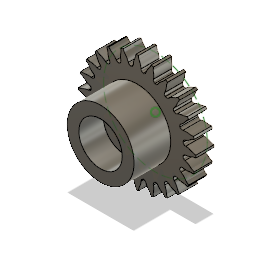
Frame Motor Gear (1) (Autodesk Fusion 360 design; units mm, degrees)
description: Spur Gear; Module: 0.708340; Num Teeth: 24; Pressure Angle: 20.000000; Backlash: 0.00 mm
Autodesk Fusion 360 part; units mm, degrees
(part 1 of 7)
sketch "Sketch1" plane through (0, 0, 0) normal (0, 0, 1) x (1, 0, 0) in component "Spur Gear (24 teeth)"
  circle A0 centre (0, 0) radius 7.5993
  circle A1 centre (0, 0) radius 0.35
extrude "Extrude1" add sketch "Sketch1" along normal blind 3 in component "Spur Gear (24 teeth)"
sketch "Sketch2" plane through (0, 0, 0) normal (0, 0, 1) x (1, 0, 0) in component "Spur Gear (24 teeth)"
  spline S0 degree 5 poles (7.9617, -0.6411) (7.9654, -0.6414) (7.9728, -0.6419) (7.9839, -0.6424) (7.9987, -0.6424) (8.0173, -0.6418) (8.0359, -0.6406) (8.0545, -0.6391) (8.0731, -0.6375) (8.0917, -0.6357) (8.1103, -0.6338) (8.129, -0.6317) (8.1476, -0.6294) (8.1663, -0.6268) (8.185, -0.6239) (8.2036, -0.6208) (8.2223, -0.6175) (8.241, -0.6141) (8.2597, -0.6105) (8.2783, -0.6068) (8.297, -0.6029) (8.3157, -0.5988) (8.3344, -0.5946) (8.3531, -0.5902) (8.3718, -0.5857) (8.3904, -0.581) (8.4091, -0.5761) (8.4278, -0.5711) (8.4465, -0.566) (8.4652, -0.5608) (8.4838, -0.5554) (8.5025, -0.5499) (8.5211, -0.5442) (8.5398, -0.5384) (8.5584, -0.5325) (8.5771, -0.5265) (8.5958, -0.5203) (8.6145, -0.514) (8.6331, -0.5076) (8.6517, -0.5011) (8.6703, -0.4944) (8.6888, -0.4876) (8.7073, -0.4807) (8.7258, -0.4737) (8.7445, -0.4666) (8.7632, -0.4593) (8.782, -0.452) (8.8008, -0.4445) (8.8194, -0.4369) (8.8377, -0.4292) (8.8558, -0.4214) (8.8737, -0.4136) (8.8918, -0.4056) (8.9103, -0.3974) (8.9293, -0.3891) (8.949, -0.3807) (8.9689, -0.3722) (8.9882, -0.3636) (9.0065, -0.3549) (9.0233, -0.3463) (9.0386, -0.3376) (9.0533, -0.3288) (9.0691, -0.3198) (9.0877, -0.3107) (9.1113, -0.3011) (9.1417, -0.291) (9.1804, -0.2805) (9.2285, -0.2692) (9.2868, -0.2574) (9.3557, -0.2448) (9.4356, -0.2316) (9.5085, -0.2204) (9.5681, -0.2117) (9.6101, -0.2058) (9.6316, -0.2028) knots 0 0 0 0 0 0 0.01428571 0.02857143 0.04285714 0.05714286 0.07142857 0.08571429 0.1 0.11428571 0.12857143 0.14285714 0.15714286 0.17142857 0.18571429 0.2 0.21428571 0.22857143 0.24285714 0.25714286 0.27142857 0.28571429 0.3 0.31428571 0.32857143 0.34285714 0.35714286 0.37142857 0.38571429 0.4 0.41428571 0.42857143 0.44285714 0.45714286 0.47142857 0.48571429 0.5 0.51428571 0.52857143 0.54285714 0.55714286 0.57142857 0.58571429 0.6 0.61428571 0.62857143 0.64285714 0.65714286 0.67142857 0.68571429 0.7 0.71428571 0.72857143 0.74285714 0.75714286 0.77142857 0.78571429 0.8 0.81428571 0.82857143 0.84285714 0.85714286 0.87142857 0.88571429 0.9 0.91428571 0.92857143 0.94285714 0.95714286 0.97142857 0.98571429 1 1 1 1 1 1
  spline S1 degree 5 poles (7.9617, 0.6411) (7.9654, 0.6414) (7.9728, 0.6419) (7.9839, 0.6424) (7.9987, 0.6424) (8.0173, 0.6418) (8.0359, 0.6406) (8.0545, 0.6391) (8.0731, 0.6375) (8.0917, 0.6357) (8.1103, 0.6338) (8.129, 0.6317) (8.1476, 0.6294) (8.1663, 0.6268) (8.185, 0.6239) (8.2036, 0.6208) (8.2223, 0.6175) (8.241, 0.6141) (8.2597, 0.6105) (8.2783, 0.6068) (8.297, 0.6029) (8.3157, 0.5988) (8.3344, 0.5946) (8.3531, 0.5902) (8.3718, 0.5857) (8.3904, 0.581) (8.4091, 0.5761) (8.4278, 0.5711) (8.4465, 0.566) (8.4652, 0.5608) (8.4838, 0.5554) (8.5025, 0.5499) (8.5211, 0.5442) (8.5398, 0.5384) (8.5584, 0.5325) (8.5771, 0.5265) (8.5958, 0.5203) (8.6145, 0.514) (8.6331, 0.5076) (8.6517, 0.5011) (8.6703, 0.4944) (8.6888, 0.4876) (8.7073, 0.4807) (8.7258, 0.4737) (8.7445, 0.4666) (8.7632, 0.4593) (8.782, 0.452) (8.8008, 0.4445) (8.8194, 0.4369) (8.8377, 0.4292) (8.8558, 0.4214) (8.8737, 0.4136) (8.8918, 0.4056) (8.9103, 0.3974) (8.9293, 0.3891) (8.949, 0.3807) (8.9689, 0.3722) (8.9882, 0.3636) (9.0065, 0.3549) (9.0233, 0.3463) (9.0386, 0.3376) (9.0533, 0.3288) (9.0691, 0.3198) (9.0877, 0.3107) (9.1113, 0.3011) (9.1417, 0.291) (9.1804, 0.2805) (9.2285, 0.2692) (9.2868, 0.2574) (9.3557, 0.2448) (9.4356, 0.2316) (9.5085, 0.2204) (9.5681, 0.2117) (9.6101, 0.2058) (9.6316, 0.2028) knots 0 0 0 0 0 0 0.01428571 0.02857143 0.04285714 0.05714286 0.07142857 0.08571429 0.1 0.11428571 0.12857143 0.14285714 0.15714286 0.17142857 0.18571429 0.2 0.21428571 0.22857143 0.24285714 0.25714286 0.27142857 0.28571429 0.3 0.31428571 0.32857143 0.34285714 0.35714286 0.37142857 0.38571429 0.4 0.41428571 0.42857143 0.44285714 0.45714286 0.47142857 0.48571429 0.5 0.51428571 0.52857143 0.54285714 0.55714286 0.57142857 0.58571429 0.6 0.61428571 0.62857143 0.64285714 0.65714286 0.67142857 0.68571429 0.7 0.71428571 0.72857143 0.74285714 0.75714286 0.77142857 0.78571429 0.8 0.81428571 0.82857143 0.84285714 0.85714286 0.87142857 0.88571429 0.9 0.91428571 0.92857143 0.94285714 0.95714286 0.97142857 0.98571429 1 1 1 1 1 1
  arc A0 (9.6316, -0.2028) -> (9.6316, 0.2028) centre (0, 0) ccw
  line L0 (7.5648, -0.61) -> (7.9617, -0.6411)
  line L1 (7.5648, 0.61) -> (7.9617, 0.6411)
  line L2 (7.5648, -0.61) -> (7.5648, 0.61)
extrude "Extrude2" add sketch "Sketch2" along normal blind 3 in component "Spur Gear (24 teeth)"
fillet "Fillet1" radius 0.4 2 edges at (7.5747, -0.6108, 1.5) (7.5747, 0.6108, 1.5) in component "Spur Gear (24 teeth)"
pattern_circular "C-Pattern1" count 24 over 360 about axis through (0, 0, 0) along (0, 0, 1) of "Extrude2", "Fillet1" in component "Spur Gear (24 teeth)"
sketch "Sketch3" plane through (0, 0, 0) normal (0, 0, 1) x (1, 0, 0) in component "Spur Gear (24 teeth)"
  circle A0 centre (0, 0) radius 8.5001 construction
sketch "Sketch1 (2)" plane through (0, 0, 3) normal (0, 0, 1) x (1, 0, 0)
  arc A0 (7.5337, -0.9958) -> (7.5348, -0.988) centre (0, 0) ccw
  arc A1 (7.9617, -0.6411) -> (7.5348, -0.988) centre (7.9314, -1.04) ccw
  spline S0 degree 5 poles (7.9617, -0.6411) (7.9654, -0.6414) (7.9728, -0.6419) (7.9839, -0.6424) (7.9987, -0.6424) (8.0173, -0.6418) (8.0359, -0.6406) (8.0545, -0.6391) (8.0731, -0.6375) (8.0917, -0.6357) (8.1103, -0.6338) (8.129, -0.6317) (8.1476, -0.6294) (8.1663, -0.6268) (8.185, -0.6239) (8.2036, -0.6208) (8.2223, -0.6175) (8.241, -0.6141) (8.2597, -0.6105) (8.2783, -0.6068) (8.297, -0.6029) (8.3157, -0.5988) (8.3344, -0.5946) (8.3531, -0.5902) (8.3718, -0.5857) (8.3904, -0.581) (8.4091, -0.5761) (8.4278, -0.5711) (8.4465, -0.566) (8.4652, -0.5608) (8.4838, -0.5554) (8.5025, -0.5499) (8.5211, -0.5442) (8.5398, -0.5384) (8.5584, -0.5325) (8.5771, -0.5265) (8.5958, -0.5203) (8.6145, -0.514) (8.6331, -0.5076) (8.6517, -0.5011) (8.6703, -0.4944) (8.6888, -0.4876) (8.7073, -0.4807) (8.7258, -0.4737) (8.7445, -0.4666) (8.7632, -0.4593) (8.782, -0.452) (8.8008, -0.4445) (8.8194, -0.4369) (8.8377, -0.4292) (8.8558, -0.4214) (8.8737, -0.4136) (8.8918, -0.4056) (8.9103, -0.3974) (8.9293, -0.3891) (8.949, -0.3807) (8.9689, -0.3722) (8.9882, -0.3636) (9.0065, -0.3549) (9.0233, -0.3463) (9.0386, -0.3376) (9.0533, -0.3288) (9.0691, -0.3198) (9.0877, -0.3107) (9.1113, -0.3011) (9.1417, -0.291) (9.1804, -0.2805) (9.2285, -0.2692) (9.2868, -0.2574) (9.3557, -0.2448) (9.4356, -0.2316) (9.5085, -0.2204) (9.5681, -0.2117) (9.6101, -0.2058) (9.6316, -0.2028) knots 0 0 0 0 0 0 0.01428571 0.02857143 0.04285714 0.05714286 0.07142857 0.08571429 0.1 0.11428571 0.12857143 0.14285714 0.15714286 0.17142857 0.18571429 0.2 0.21428571 0.22857143 0.24285714 0.25714286 0.27142857 0.28571429 0.3 0.31428571 0.32857143 0.34285714 0.35714286 0.37142857 0.38571429 0.4 0.41428571 0.42857143 0.44285714 0.45714286 0.47142857 0.48571429 0.5 0.51428571 0.52857143 0.54285714 0.55714286 0.57142857 0.58571429 0.6 0.61428571 0.62857143 0.64285714 0.65714286 0.67142857 0.68571429 0.7 0.71428571 0.72857143 0.74285714 0.75714286 0.77142857 0.78571429 0.8 0.81428571 0.82857143 0.84285714 0.85714286 0.87142857 0.88571429 0.9 0.91428571 0.92857143 0.94285714 0.95714286 0.97142857 0.98571429 1 1 1 1 1 1
  arc A2 (9.6316, -0.2028) -> (9.6316, 0.2028) centre (0, 0) ccw
  spline S1 degree 5 poles (9.6316, 0.2028) (9.6101, 0.2058) (9.5681, 0.2117) (9.5085, 0.2204) (9.4356, 0.2316) (9.3557, 0.2448) (9.2868, 0.2574) (9.2285, 0.2692) (9.1804, 0.2805) (9.1417, 0.291) (9.1113, 0.3011) (9.0877, 0.3107) (9.0691, 0.3198) (9.0533, 0.3288) (9.0386, 0.3376) (9.0233, 0.3463) (9.0065, 0.3549) (8.9882, 0.3636) (8.9689, 0.3722) (8.949, 0.3807) (8.9293, 0.3891) (8.9103, 0.3974) (8.8918, 0.4056) (8.8737, 0.4136) (8.8558, 0.4214) (8.8377, 0.4292) (8.8194, 0.4369) (8.8008, 0.4445) (8.782, 0.452) (8.7632, 0.4593) (8.7445, 0.4666) (8.7258, 0.4737) (8.7073, 0.4807) (8.6888, 0.4876) (8.6703, 0.4944) (8.6517, 0.5011) (8.6331, 0.5076) (8.6145, 0.514) (8.5958, 0.5203) (8.5771, 0.5265) (8.5584, 0.5325) (8.5398, 0.5384) (8.5211, 0.5442) (8.5025, 0.5499) (8.4838, 0.5554) (8.4652, 0.5608) (8.4465, 0.566) (8.4278, 0.5711) (8.4091, 0.5761) (8.3904, 0.581) (8.3718, 0.5857) (8.3531, 0.5902) (8.3344, 0.5946) (8.3157, 0.5988) (8.297, 0.6029) (8.2783, 0.6068) (8.2597, 0.6105) (8.241, 0.6141) (8.2223, 0.6175) (8.2036, 0.6208) (8.185, 0.6239) (8.1663, 0.6268) (8.1476, 0.6294) (8.129, 0.6317) (8.1103, 0.6338) (8.0917, 0.6357) (8.0731, 0.6375) (8.0545, 0.6391) (8.0359, 0.6406) (8.0173, 0.6418) (7.9987, 0.6424) (7.9839, 0.6424) (7.9728, 0.6419) (7.9654, 0.6414) (7.9617, 0.6411) knots -1 -1 -1 -1 -1 -1 -0.98571429 -0.97142857 -0.95714286 -0.94285714 -0.92857143 -0.91428571 -0.9 -0.88571429 -0.87142857 -0.85714286 -0.84285714 -0.82857143 -0.81428571 -0.8 -0.78571429 -0.77142857 -0.75714286 -0.74285714 -0.72857143 -0.71428571 -0.7 -0.68571429 -0.67142857 -0.65714286 -0.64285714 -0.62857143 -0.61428571 -0.6 -0.58571429 -0.57142857 -0.55714286 -0.54285714 -0.52857143 -0.51428571 -0.5 -0.48571429 -0.47142857 -0.45714286 -0.44285714 -0.42857143 -0.41428571 -0.4 -0.38571429 -0.37142857 -0.35714286 -0.34285714 -0.32857143 -0.31428571 -0.3 -0.28571429 -0.27142857 -0.25714286 -0.24285714 -0.22857143 -0.21428571 -0.2 -0.18571429 -0.17142857 -0.15714286 -0.14285714 -0.12857143 -0.11428571 -0.1 -0.08571429 -0.07142857 -0.05714286 -0.04285714 -0.02857143 -0.01428571 0 0 0 0 0 0
  arc A3 (7.5348, 0.988) -> (7.9617, 0.6411) centre (7.9314, 1.04) ccw
  arc A4 (7.5348, 0.988) -> (7.5337, 0.9958) centre (0, 0) ccw
  arc A5 (7.8563, 1.4413) -> (7.5337, 0.9958) centre (7.9303, 1.0482) ccw
  spline S2 degree 5 poles (7.8563, 1.4413) (7.86, 1.442) (7.8673, 1.4435) (7.8781, 1.4459) (7.8924, 1.4497) (7.9102, 1.4551) (7.9278, 1.461) (7.9454, 1.4673) (7.963, 1.4737) (7.9805, 1.4802) (7.998, 1.4869) (8.0155, 1.4937) (8.0329, 1.5008) (8.0503, 1.5082) (8.0675, 1.5158) (8.0848, 1.5236) (8.102, 1.5316) (8.1191, 1.5398) (8.1362, 1.5481) (8.1533, 1.5565) (8.1703, 1.5651) (8.1873, 1.5739) (8.2043, 1.5828) (8.2212, 1.5918) (8.2381, 1.6011) (8.2549, 1.6104) (8.2717, 1.6199) (8.2885, 1.6296) (8.3052, 1.6394) (8.3219, 1.6493) (8.3385, 1.6593) (8.3551, 1.6695) (8.3716, 1.6797) (8.3881, 1.6902) (8.4046, 1.7007) (8.4211, 1.7114) (8.4375, 1.7222) (8.454, 1.7331) (8.4703, 1.7441) (8.4866, 1.7552) (8.5028, 1.7665) (8.5189, 1.7778) (8.535, 1.7892) (8.5511, 1.8008) (8.5673, 1.8125) (8.5835, 1.8244) (8.5998, 1.8364) (8.616, 1.8485) (8.632, 1.8606) (8.6477, 1.8728) (8.6631, 1.885) (8.6784, 1.8972) (8.6938, 1.9096) (8.7095, 1.9223) (8.7258, 1.9352) (8.7426, 1.9484) (8.7596, 1.9618) (8.7761, 1.9751) (8.7915, 1.9882) (8.8054, 2.0009) (8.818, 2.0133) (8.8299, 2.0256) (8.8428, 2.0383) (8.8585, 2.052) (8.8788, 2.0674) (8.9055, 2.0849) (8.9402, 2.1052) (8.9838, 2.1285) (9.037, 2.155) (9.1003, 2.185) (9.1741, 2.2184) (9.2415, 2.2481) (9.2968, 2.2719) (9.3359, 2.2885) (9.3559, 2.297) knots 0 0 0 0 0 0 0.01428571 0.02857143 0.04285714 0.05714286 0.07142857 0.08571429 0.1 0.11428571 0.12857143 0.14285714 0.15714286 0.17142857 0.18571429 0.2 0.21428571 0.22857143 0.24285714 0.25714286 0.27142857 0.28571429 0.3 0.31428571 0.32857143 0.34285714 0.35714286 0.37142857 0.38571429 0.4 0.41428571 0.42857143 0.44285714 0.45714286 0.47142857 0.48571429 0.5 0.51428571 0.52857143 0.54285714 0.55714286 0.57142857 0.58571429 0.6 0.61428571 0.62857143 0.64285714 0.65714286 0.67142857 0.68571429 0.7 0.71428571 0.72857143 0.74285714 0.75714286 0.77142857 0.78571429 0.8 0.81428571 0.82857143 0.84285714 0.85714286 0.87142857 0.88571429 0.9 0.91428571 0.92857143 0.94285714 0.95714286 0.97142857 0.98571429 1 1 1 1 1 1
  arc A6 (9.3559, 2.297) -> (9.2509, 2.6887) centre (0, 0) ccw
  spline S3 degree 5 poles (9.2509, 2.6887) (9.2293, 2.686) (9.1873, 2.6809) (9.1274, 2.6739) (9.0542, 2.6658) (8.9736, 2.6579) (8.9037, 2.6522) (8.8444, 2.6486) (8.795, 2.647) (8.7549, 2.6472) (8.7229, 2.649) (8.6977, 2.6521) (8.6773, 2.6562) (8.6598, 2.6608) (8.6432, 2.6654) (8.6262, 2.6699) (8.6078, 2.6739) (8.5879, 2.6775) (8.5669, 2.6808) (8.5455, 2.6839) (8.5244, 2.687) (8.5038, 2.69) (8.4838, 2.6931) (8.4643, 2.6962) (8.445, 2.6991) (8.4255, 2.702) (8.4058, 2.7047) (8.3859, 2.7072) (8.3658, 2.7095) (8.3457, 2.7118) (8.3257, 2.7139) (8.3059, 2.716) (8.2861, 2.718) (8.2665, 2.7198) (8.2469, 2.7216) (8.2272, 2.7232) (8.2076, 2.7247) (8.1879, 2.7261) (8.1682, 2.7273) (8.1486, 2.7285) (8.129, 2.7295) (8.1094, 2.7303) (8.0899, 2.7311) (8.0704, 2.7317) (8.051, 2.7322) (8.0316, 2.7326) (8.0122, 2.7329) (7.9928, 2.733) (7.9735, 2.7329) (7.9542, 2.7328) (7.9349, 2.7325) (7.9157, 2.732) (7.8965, 2.7314) (7.8774, 2.7307) (7.8583, 2.7297) (7.8392, 2.7287) (7.8202, 2.7275) (7.8012, 2.7261) (7.7823, 2.7246) (7.7634, 2.7229) (7.7446, 2.7211) (7.7258, 2.719) (7.7071, 2.7167) (7.6885, 2.7141) (7.6699, 2.7113) (7.6514, 2.7084) (7.633, 2.7052) (7.6146, 2.702) (7.5962, 2.6986) (7.578, 2.6949) (7.5599, 2.6908) (7.5456, 2.6869) (7.535, 2.6835) (7.528, 2.6812) (7.5245, 2.6799) knots -1 -1 -1 -1 -1 -1 -0.98571429 -0.97142857 -0.95714286 -0.94285714 -0.92857143 -0.91428571 -0.9 -0.88571429 -0.87142857 -0.85714286 -0.84285714 -0.82857143 -0.81428571 -0.8 -0.78571429 -0.77142857 -0.75714286 -0.74285714 -0.72857143 -0.71428571 -0.7 -0.68571429 -0.67142857 -0.65714286 -0.64285714 -0.62857143 -0.61428571 -0.6 -0.58571429 -0.57142857 -0.55714286 -0.54285714 -0.52857143 -0.51428571 -0.5 -0.48571429 -0.47142857 -0.45714286 -0.44285714 -0.42857143 -0.41428571 -0.4 -0.38571429 -0.37142857 -0.35714286 -0.34285714 -0.32857143 -0.31428571 -0.3 -0.28571429 -0.27142857 -0.25714286 -0.24285714 -0.22857143 -0.21428571 -0.2 -0.18571429 -0.17142857 -0.15714286 -0.14285714 -0.12857143 -0.11428571 -0.1 -0.08571429 -0.07142857 -0.05714286 -0.04285714 -0.02857143 -0.01428571 0 0 0 0 0 0
  arc A7 (7.0223, 2.9045) -> (7.5245, 2.6799) centre (7.392, 3.0573) ccw
  arc A8 (7.0223, 2.9045) -> (7.0193, 2.9118) centre (0, 0) ccw
  arc A9 (7.2156, 3.4256) -> (7.0193, 2.9118) centre (7.3888, 3.065) ccw
  spline S4 degree 5 poles (7.2156, 3.4256) (7.2189, 3.4272) (7.2256, 3.4305) (7.2354, 3.4356) (7.2483, 3.443) (7.264, 3.4528) (7.2796, 3.4631) (7.2949, 3.4737) (7.3102, 3.4844) (7.3255, 3.4953) (7.3407, 3.5063) (7.3558, 3.5174) (7.3707, 3.5288) (7.3856, 3.5403) (7.4003, 3.5521) (7.415, 3.5642) (7.4295, 3.5763) (7.4439, 3.5887) (7.4583, 3.6011) (7.4726, 3.6137) (7.4869, 3.6264) (7.501, 3.6393) (7.5151, 3.6523) (7.5291, 3.6654) (7.543, 3.6787) (7.5568, 3.6921) (7.5706, 3.7056) (7.5843, 3.7193) (7.5979, 3.7331) (7.6114, 3.7469) (7.6249, 3.7609) (7.6383, 3.775) (7.6516, 3.7892) (7.6649, 3.8036) (7.6781, 3.818) (7.6912, 3.8326) (7.7043, 3.8473) (7.7173, 3.8621) (7.7303, 3.877) (7.7431, 3.8919) (7.7559, 3.907) (7.7685, 3.9221) (7.7811, 3.9373) (7.7936, 3.9526) (7.8062, 3.9681) (7.8188, 3.9838) (7.8315, 3.9996) (7.844, 4.0155) (7.8563, 4.0313) (7.8683, 4.0472) (7.8801, 4.0629) (7.8916, 4.0787) (7.9033, 4.0947) (7.9152, 4.111) (7.9276, 4.1277) (7.9404, 4.1448) (7.9534, 4.1621) (7.9659, 4.1792) (7.9773, 4.1959) (7.9875, 4.2118) (7.9964, 4.227) (8.0048, 4.2419) (8.014, 4.2575) (8.0255, 4.2748) (8.0412, 4.2949) (8.0625, 4.3188) (8.0907, 4.3473) (8.1268, 4.3811) (8.1713, 4.4205) (8.2247, 4.4658) (8.2873, 4.5173) (8.3448, 4.5634) (8.3921, 4.6007) (8.4254, 4.6268) (8.4426, 4.6402) knots 0 0 0 0 0 0 0.01428571 0.02857143 0.04285714 0.05714286 0.07142857 0.08571429 0.1 0.11428571 0.12857143 0.14285714 0.15714286 0.17142857 0.18571429 0.2 0.21428571 0.22857143 0.24285714 0.25714286 0.27142857 0.28571429 0.3 0.31428571 0.32857143 0.34285714 0.35714286 0.37142857 0.38571429 0.4 0.41428571 0.42857143 0.44285714 0.45714286 0.47142857 0.48571429 0.5 0.51428571 0.52857143 0.54285714 0.55714286 0.57142857 0.58571429 0.6 0.61428571 0.62857143 0.64285714 0.65714286 0.67142857 0.68571429 0.7 0.71428571 0.72857143 0.74285714 0.75714286 0.77142857 0.78571429 0.8 0.81428571 0.82857143 0.84285714 0.85714286 0.87142857 0.88571429 0.9 0.91428571 0.92857143 0.94285714 0.95714286 0.97142857 0.98571429 1 1 1 1 1 1
  arc A10 (8.4426, 4.6402) -> (8.2398, 4.9914) centre (0, 0) ccw
  spline S5 degree 5 poles (8.2398, 4.9914) (8.2197, 4.9832) (8.1803, 4.9674) (8.1244, 4.9451) (8.0557, 4.9184) (7.9799, 4.8899) (7.9139, 4.8663) (7.8575, 4.8474) (7.8103, 4.8331) (7.7714, 4.8229) (7.7401, 4.8164) (7.7149, 4.8129) (7.6941, 4.8115) (7.676, 4.8114) (7.6589, 4.8116) (7.6412, 4.8115) (7.6224, 4.8106) (7.6023, 4.809) (7.5812, 4.8068) (7.5597, 4.8042) (7.5385, 4.8017) (7.5178, 4.7993) (7.4977, 4.7971) (7.4781, 4.795) (7.4586, 4.7929) (7.4391, 4.7906) (7.4194, 4.7881) (7.3995, 4.7854) (7.3795, 4.7824) (7.3595, 4.7794) (7.3396, 4.7763) (7.3199, 4.7732) (7.3003, 4.77) (7.2809, 4.7667) (7.2615, 4.7633) (7.2421, 4.7598) (7.2227, 4.7561) (7.2033, 4.7524) (7.184, 4.7485) (7.1647, 4.7445) (7.1455, 4.7404) (7.1264, 4.7362) (7.1074, 4.7319) (7.0884, 4.7274) (7.0695, 4.7229) (7.0507, 4.7182) (7.0319, 4.7134) (7.0131, 4.7085) (6.9945, 4.7035) (6.9758, 4.6983) (6.9573, 4.6931) (6.9389, 4.6877) (6.9205, 4.6821) (6.9022, 4.6764) (6.884, 4.6706) (6.8659, 4.6646) (6.8478, 4.6585) (6.8299, 4.6523) (6.8119, 4.646) (6.7941, 4.6395) (6.7764, 4.6328) (6.7588, 4.626) (6.7414, 4.6189) (6.724, 4.6116) (6.7068, 4.6041) (6.6897, 4.5964) (6.6727, 4.5886) (6.6558, 4.5807) (6.6389, 4.5727) (6.6223, 4.5644) (6.6059, 4.5557) (6.5931, 4.5482) (6.5837, 4.5423) (6.5775, 4.5382) (6.5745, 4.5361) knots -1 -1 -1 -1 -1 -1 -0.98571429 -0.97142857 -0.95714286 -0.94285714 -0.92857143 -0.91428571 -0.9 -0.88571429 -0.87142857 -0.85714286 -0.84285714 -0.82857143 -0.81428571 -0.8 -0.78571429 -0.77142857 -0.75714286 -0.74285714 -0.72857143 -0.71428571 -0.7 -0.68571429 -0.67142857 -0.65714286 -0.64285714 -0.62857143 -0.61428571 -0.6 -0.58571429 -0.57142857 -0.55714286 -0.54285714 -0.52857143 -0.51428571 -0.5 -0.48571429 -0.47142857 -0.45714286 -0.44285714 -0.42857143 -0.41428571 -0.4 -0.38571429 -0.37142857 -0.35714286 -0.34285714 -0.32857143 -0.31428571 -0.3 -0.28571429 -0.27142857 -0.25714286 -0.24285714 -0.22857143 -0.21428571 -0.2 -0.18571429 -0.17142857 -0.15714286 -0.14285714 -0.12857143 -0.11428571 -0.1 -0.08571429 -0.07142857 -0.05714286 -0.04285714 -0.02857143 -0.01428571 0 0 0 0 0 0
  arc A11 (6.0313, 4.623) -> (6.5745, 4.5361) centre (6.3488, 4.8663) ccw
  arc A12 (6.0313, 4.623) -> (6.0265, 4.6293) centre (0, 0) ccw
  arc A13 (6.0831, 5.1764) -> (6.0265, 4.6293) centre (6.3437, 4.873) ccw
  spline S6 degree 5 poles (6.0831, 5.1764) (6.0859, 5.1788) (6.0915, 5.1837) (6.0997, 5.1912) (6.1102, 5.2017) (6.1229, 5.2153) (6.1352, 5.2292) (6.1473, 5.2434) (6.1593, 5.2577) (6.1712, 5.2722) (6.183, 5.2867) (6.1947, 5.3014) (6.2063, 5.3162) (6.2176, 5.3312) (6.2288, 5.3465) (6.2398, 5.3618) (6.2507, 5.3774) (6.2615, 5.393) (6.2721, 5.4088) (6.2827, 5.4246) (6.2932, 5.4406) (6.3035, 5.4567) (6.3137, 5.4729) (6.3239, 5.4892) (6.3338, 5.5056) (6.3437, 5.5221) (6.3535, 5.5388) (6.3632, 5.5555) (6.3728, 5.5723) (6.3823, 5.5892) (6.3917, 5.6062) (6.401, 5.6233) (6.4102, 5.6405) (6.4193, 5.6578) (6.4283, 5.6752) (6.4372, 5.6926) (6.446, 5.7102) (6.4548, 5.7279) (6.4635, 5.7456) (6.472, 5.7634) (6.4804, 5.7812) (6.4887, 5.7991) (6.4969, 5.817) (6.5051, 5.8351) (6.5132, 5.8533) (6.5213, 5.8717) (6.5294, 5.8902) (6.5374, 5.9088) (6.5452, 5.9273) (6.5527, 5.9457) (6.56, 5.964) (6.5671, 5.9822) (6.5742, 6.0007) (6.5815, 6.0195) (6.5892, 6.0388) (6.5971, 6.0587) (6.6051, 6.0788) (6.6128, 6.0986) (6.6195, 6.1176) (6.6253, 6.1356) (6.6299, 6.1525) (6.6342, 6.1692) (6.639, 6.1866) (6.6457, 6.2063) (6.6556, 6.2298) (6.67, 6.2584) (6.6898, 6.2932) (6.7159, 6.3352) (6.7487, 6.3848) (6.7886, 6.4424) (6.8358, 6.5083) (6.8793, 6.5676) (6.9154, 6.6159) (6.9408, 6.6498) (6.9539, 6.6672) knots 0 0 0 0 0 0 0.01428571 0.02857143 0.04285714 0.05714286 0.07142857 0.08571429 0.1 0.11428571 0.12857143 0.14285714 0.15714286 0.17142857 0.18571429 0.2 0.21428571 0.22857143 0.24285714 0.25714286 0.27142857 0.28571429 0.3 0.31428571 0.32857143 0.34285714 0.35714286 0.37142857 0.38571429 0.4 0.41428571 0.42857143 0.44285714 0.45714286 0.47142857 0.48571429 0.5 0.51428571 0.52857143 0.54285714 0.55714286 0.57142857 0.58571429 0.6 0.61428571 0.62857143 0.64285714 0.65714286 0.67142857 0.68571429 0.7 0.71428571 0.72857143 0.74285714 0.75714286 0.77142857 0.78571429 0.8 0.81428571 0.82857143 0.84285714 0.85714286 0.87142857 0.88571429 0.9 0.91428571 0.92857143 0.94285714 0.95714286 0.97142857 0.98571429 1 1 1 1 1 1
  arc A14 (6.9539, 6.6672) -> (6.6672, 6.9539) centre (0, 0) ccw
  spline S7 degree 5 poles (6.6672, 6.9539) (6.6498, 6.9408) (6.6159, 6.9154) (6.5676, 6.8793) (6.5083, 6.8358) (6.4424, 6.7886) (6.3848, 6.7487) (6.3352, 6.7159) (6.2932, 6.6898) (6.2584, 6.67) (6.2298, 6.6556) (6.2063, 6.6457) (6.1866, 6.639) (6.1692, 6.6342) (6.1525, 6.6299) (6.1356, 6.6253) (6.1176, 6.6195) (6.0986, 6.6128) (6.0788, 6.6051) (6.0587, 6.5971) (6.0388, 6.5892) (6.0195, 6.5815) (6.0007, 6.5742) (5.9822, 6.5671) (5.964, 6.56) (5.9457, 6.5527) (5.9273, 6.5452) (5.9088, 6.5374) (5.8902, 6.5294) (5.8717, 6.5213) (5.8533, 6.5132) (5.8351, 6.5051) (5.817, 6.4969) (5.7991, 6.4887) (5.7812, 6.4804) (5.7634, 6.472) (5.7456, 6.4635) (5.7279, 6.4548) (5.7102, 6.446) (5.6926, 6.4372) (5.6752, 6.4283) (5.6578, 6.4193) (5.6405, 6.4102) (5.6233, 6.401) (5.6062, 6.3917) (5.5892, 6.3823) (5.5723, 6.3728) (5.5555, 6.3632) (5.5388, 6.3535) (5.5221, 6.3437) (5.5056, 6.3338) (5.4892, 6.3239) (5.4729, 6.3137) (5.4567, 6.3035) (5.4406, 6.2932) (5.4246, 6.2827) (5.4088, 6.2721) (5.393, 6.2615) (5.3774, 6.2507) (5.3618, 6.2398) (5.3465, 6.2288) (5.3312, 6.2176) (5.3162, 6.2063) (5.3014, 6.1947) (5.2867, 6.183) (5.2722, 6.1712) (5.2577, 6.1593) (5.2434, 6.1473) (5.2292, 6.1352) (5.2153, 6.1229) (5.2017, 6.1102) (5.1912, 6.0997) (5.1837, 6.0915) (5.1788, 6.0859) (5.1764, 6.0831) knots -1 -1 -1 -1 -1 -1 -0.98571429 -0.97142857 -0.95714286 -0.94285714 -0.92857143 -0.91428571 -0.9 -0.88571429 -0.87142857 -0.85714286 -0.84285714 -0.82857143 -0.81428571 -0.8 -0.78571429 -0.77142857 -0.75714286 -0.74285714 -0.72857143 -0.71428571 -0.7 -0.68571429 -0.67142857 -0.65714286 -0.64285714 -0.62857143 -0.61428571 -0.6 -0.58571429 -0.57142857 -0.55714286 -0.54285714 -0.52857143 -0.51428571 -0.5 -0.48571429 -0.47142857 -0.45714286 -0.44285714 -0.42857143 -0.41428571 -0.4 -0.38571429 -0.37142857 -0.35714286 -0.34285714 -0.32857143 -0.31428571 -0.3 -0.28571429 -0.27142857 -0.25714286 -0.24285714 -0.22857143 -0.21428571 -0.2 -0.18571429 -0.17142857 -0.15714286 -0.14285714 -0.12857143 -0.11428571 -0.1 -0.08571429 -0.07142857 -0.05714286 -0.04285714 -0.02857143 -0.01428571 0 0 0 0 0 0
  arc A15 (4.6293, 6.0265) -> (5.1764, 6.0831) centre (4.873, 6.3437) ccw
  arc A16 (4.6293, 6.0265) -> (4.623, 6.0313) centre (0, 0) ccw
  arc A17 (4.5361, 6.5745) -> (4.623, 6.0313) centre (4.8663, 6.3488) ccw
  spline S8 degree 5 poles (4.5361, 6.5745) (4.5382, 6.5775) (4.5423, 6.5837) (4.5482, 6.5931) (4.5557, 6.6059) (4.5644, 6.6223) (4.5727, 6.6389) (4.5807, 6.6558) (4.5886, 6.6727) (4.5964, 6.6897) (4.6041, 6.7068) (4.6116, 6.724) (4.6189, 6.7414) (4.626, 6.7588) (4.6328, 6.7764) (4.6395, 6.7941) (4.646, 6.8119) (4.6523, 6.8299) (4.6585, 6.8478) (4.6646, 6.8659) (4.6706, 6.884) (4.6764, 6.9022) (4.6821, 6.9205) (4.6877, 6.9389) (4.6931, 6.9573) (4.6983, 6.9758) (4.7035, 6.9945) (4.7085, 7.0131) (4.7134, 7.0319) (4.7182, 7.0507) (4.7229, 7.0695) (4.7274, 7.0884) (4.7319, 7.1074) (4.7362, 7.1264) (4.7404, 7.1455) (4.7445, 7.1647) (4.7485, 7.184) (4.7524, 7.2033) (4.7561, 7.2227) (4.7598, 7.2421) (4.7633, 7.2615) (4.7667, 7.2809) (4.77, 7.3003) (4.7732, 7.3199) (4.7763, 7.3396) (4.7794, 7.3595) (4.7824, 7.3795) (4.7854, 7.3995) (4.7881, 7.4194) (4.7906, 7.4391) (4.7929, 7.4586) (4.795, 7.4781) (4.7971, 7.4977) (4.7993, 7.5178) (4.8017, 7.5385) (4.8042, 7.5597) (4.8068, 7.5812) (4.809, 7.6023) (4.8106, 7.6224) (4.8115, 7.6412) (4.8116, 7.6589) (4.8114, 7.676) (4.8115, 7.6941) (4.8129, 7.7149) (4.8164, 7.7401) (4.8229, 7.7714) (4.8331, 7.8103) (4.8474, 7.8575) (4.8663, 7.9139) (4.8899, 7.9799) (4.9184, 8.0557) (4.9451, 8.1244) (4.9674, 8.1803) (4.9832, 8.2197) (4.9914, 8.2398) knots 0 0 0 0 0 0 0.01428571 0.02857143 0.04285714 0.05714286 0.07142857 0.08571429 0.1 0.11428571 0.12857143 0.14285714 0.15714286 0.17142857 0.18571429 0.2 0.21428571 0.22857143 0.24285714 0.25714286 0.27142857 0.28571429 0.3 0.31428571 0.32857143 0.34285714 0.35714286 0.37142857 0.38571429 0.4 0.41428571 0.42857143 0.44285714 0.45714286 0.47142857 0.48571429 0.5 0.51428571 0.52857143 0.54285714 0.55714286 0.57142857 0.58571429 0.6 0.61428571 0.62857143 0.64285714 0.65714286 0.67142857 0.68571429 0.7 0.71428571 0.72857143 0.74285714 0.75714286 0.77142857 0.78571429 0.8 0.81428571 0.82857143 0.84285714 0.85714286 0.87142857 0.88571429 0.9 0.91428571 0.92857143 0.94285714 0.95714286 0.97142857 0.98571429 1 1 1 1 1 1
  arc A18 (4.9914, 8.2398) -> (4.6402, 8.4426) centre (0, 0) ccw
  spline S9 degree 5 poles (4.6402, 8.4426) (4.6268, 8.4254) (4.6007, 8.3921) (4.5634, 8.3448) (4.5173, 8.2873) (4.4658, 8.2247) (4.4205, 8.1713) (4.3811, 8.1268) (4.3473, 8.0907) (4.3188, 8.0625) (4.2949, 8.0412) (4.2748, 8.0255) (4.2575, 8.014) (4.2419, 8.0048) (4.227, 7.9964) (4.2118, 7.9875) (4.1959, 7.9773) (4.1792, 7.9659) (4.1621, 7.9534) (4.1448, 7.9404) (4.1277, 7.9276) (4.111, 7.9152) (4.0947, 7.9033) (4.0787, 7.8916) (4.0629, 7.8801) (4.0472, 7.8683) (4.0313, 7.8563) (4.0155, 7.844) (3.9996, 7.8315) (3.9838, 7.8188) (3.9681, 7.8062) (3.9526, 7.7936) (3.9373, 7.7811) (3.9221, 7.7685) (3.907, 7.7559) (3.8919, 7.7431) (3.877, 7.7303) (3.8621, 7.7173) (3.8473, 7.7043) (3.8326, 7.6912) (3.818, 7.6781) (3.8036, 7.6649) (3.7892, 7.6516) (3.775, 7.6383) (3.7609, 7.6249) (3.7469, 7.6114) (3.7331, 7.5979) (3.7193, 7.5843) (3.7056, 7.5706) (3.6921, 7.5568) (3.6787, 7.543) (3.6654, 7.5291) (3.6523, 7.5151) (3.6393, 7.501) (3.6264, 7.4869) (3.6137, 7.4726) (3.6011, 7.4583) (3.5887, 7.4439) (3.5763, 7.4295) (3.5642, 7.415) (3.5521, 7.4003) (3.5403, 7.3856) (3.5288, 7.3707) (3.5174, 7.3558) (3.5063, 7.3407) (3.4953, 7.3255) (3.4844, 7.3102) (3.4737, 7.2949) (3.4631, 7.2796) (3.4528, 7.264) (3.443, 7.2483) (3.4356, 7.2354) (3.4305, 7.2256) (3.4272, 7.2189) (3.4256, 7.2156) knots -1 -1 -1 -1 -1 -1 -0.98571429 -0.97142857 -0.95714286 -0.94285714 -0.92857143 -0.91428571 -0.9 -0.88571429 -0.87142857 -0.85714286 -0.84285714 -0.82857143 -0.81428571 -0.8 -0.78571429 -0.77142857 -0.75714286 -0.74285714 -0.72857143 -0.71428571 -0.7 -0.68571429 -0.67142857 -0.65714286 -0.64285714 -0.62857143 -0.61428571 -0.6 -0.58571429 -0.57142857 -0.55714286 -0.54285714 -0.52857143 -0.51428571 -0.5 -0.48571429 -0.47142857 -0.45714286 -0.44285714 -0.42857143 -0.41428571 -0.4 -0.38571429 -0.37142857 -0.35714286 -0.34285714 -0.32857143 -0.31428571 -0.3 -0.28571429 -0.27142857 -0.25714286 -0.24285714 -0.22857143 -0.21428571 -0.2 -0.18571429 -0.17142857 -0.15714286 -0.14285714 -0.12857143 -0.11428571 -0.1 -0.08571429 -0.07142857 -0.05714286 -0.04285714 -0.02857143 -0.01428571 0 0 0 0 0 0
  arc A19 (2.9118, 7.0193) -> (3.4256, 7.2156) centre (3.065, 7.3888) ccw
  arc A20 (2.9118, 7.0193) -> (2.9045, 7.0223) centre (0, 0) ccw
  arc A21 (2.6799, 7.5245) -> (2.9045, 7.0223) centre (3.0573, 7.392) ccw
  spline S10 degree 5 poles (2.6799, 7.5245) (2.6812, 7.528) (2.6835, 7.535) (2.6869, 7.5456) (2.6908, 7.5599) (2.6949, 7.578) (2.6986, 7.5962) (2.702, 7.6146) (2.7052, 7.633) (2.7084, 7.6514) (2.7113, 7.6699) (2.7141, 7.6885) (2.7167, 7.7071) (2.719, 7.7258) (2.7211, 7.7446) (2.7229, 7.7634) (2.7246, 7.7823) (2.7261, 7.8012) (2.7275, 7.8202) (2.7287, 7.8392) (2.7297, 7.8583) (2.7307, 7.8774) (2.7314, 7.8965) (2.732, 7.9157) (2.7325, 7.9349) (2.7328, 7.9542) (2.7329, 7.9735) (2.733, 7.9928) (2.7329, 8.0122) (2.7326, 8.0316) (2.7322, 8.051) (2.7317, 8.0704) (2.7311, 8.0899) (2.7303, 8.1094) (2.7295, 8.129) (2.7285, 8.1486) (2.7273, 8.1682) (2.7261, 8.1879) (2.7247, 8.2076) (2.7232, 8.2272) (2.7216, 8.2469) (2.7198, 8.2665) (2.718, 8.2861) (2.716, 8.3059) (2.7139, 8.3257) (2.7118, 8.3457) (2.7095, 8.3658) (2.7072, 8.3859) (2.7047, 8.4058) (2.702, 8.4255) (2.6991, 8.445) (2.6962, 8.4643) (2.6931, 8.4838) (2.69, 8.5038) (2.687, 8.5244) (2.6839, 8.5455) (2.6808, 8.5669) (2.6775, 8.5879) (2.6739, 8.6078) (2.6699, 8.6262) (2.6654, 8.6432) (2.6608, 8.6598) (2.6562, 8.6773) (2.6521, 8.6977) (2.649, 8.7229) (2.6472, 8.7549) (2.647, 8.795) (2.6486, 8.8444) (2.6522, 8.9037) (2.6579, 8.9736) (2.6658, 9.0542) (2.6739, 9.1274) (2.6809, 9.1873) (2.686, 9.2293) (2.6887, 9.2509) knots 0 0 0 0 0 0 0.01428571 0.02857143 0.04285714 0.05714286 0.07142857 0.08571429 0.1 0.11428571 0.12857143 0.14285714 0.15714286 0.17142857 0.18571429 0.2 0.21428571 0.22857143 0.24285714 0.25714286 0.27142857 0.28571429 0.3 0.31428571 0.32857143 0.34285714 0.35714286 0.37142857 0.38571429 0.4 0.41428571 0.42857143 0.44285714 0.45714286 0.47142857 0.48571429 0.5 0.51428571 0.52857143 0.54285714 0.55714286 0.57142857 0.58571429 0.6 0.61428571 0.62857143 0.64285714 0.65714286 0.67142857 0.68571429 0.7 0.71428571 0.72857143 0.74285714 0.75714286 0.77142857 0.78571429 0.8 0.81428571 0.82857143 0.84285714 0.85714286 0.87142857 0.88571429 0.9 0.91428571 0.92857143 0.94285714 0.95714286 0.97142857 0.98571429 1 1 1 1 1 1
  arc A22 (2.6887, 9.2509) -> (2.297, 9.3559) centre (0, 0) ccw
  spline S11 degree 5 poles (2.297, 9.3559) (2.2885, 9.3359) (2.2719, 9.2968) (2.2481, 9.2415) (2.2184, 9.1741) (2.185, 9.1003) (2.155, 9.037) (2.1285, 8.9838) (2.1052, 8.9402) (2.0849, 8.9055) (2.0674, 8.8788) (2.052, 8.8585) (2.0383, 8.8428) (2.0256, 8.8299) (2.0133, 8.818) (2.0009, 8.8054) (1.9882, 8.7915) (1.9751, 8.7761) (1.9618, 8.7596) (1.9484, 8.7426) (1.9352, 8.7258) (1.9223, 8.7095) (1.9096, 8.6938) (1.8972, 8.6784) (1.885, 8.6631) (1.8728, 8.6477) (1.8606, 8.632) (1.8485, 8.616) (1.8364, 8.5998) (1.8244, 8.5835) (1.8125, 8.5673) (1.8008, 8.5511) (1.7892, 8.535) (1.7778, 8.5189) (1.7665, 8.5028) (1.7552, 8.4866) (1.7441, 8.4703) (1.7331, 8.454) (1.7222, 8.4375) (1.7114, 8.4211) (1.7007, 8.4046) (1.6902, 8.3881) (1.6797, 8.3716) (1.6695, 8.3551) (1.6593, 8.3385) (1.6493, 8.3219) (1.6394, 8.3052) (1.6296, 8.2885) (1.6199, 8.2717) (1.6104, 8.2549) (1.6011, 8.2381) (1.5918, 8.2212) (1.5828, 8.2043) (1.5739, 8.1873) (1.5651, 8.1703) (1.5565, 8.1533) (1.5481, 8.1362) (1.5398, 8.1191) (1.5316, 8.102) (1.5236, 8.0848) (1.5158, 8.0675) (1.5082, 8.0503) (1.5008, 8.0329) (1.4937, 8.0155) (1.4869, 7.998) (1.4802, 7.9805) (1.4737, 7.963) (1.4673, 7.9454) (1.461, 7.9278) (1.4551, 7.9102) (1.4497, 7.8924) (1.4459, 7.8781) (1.4435, 7.8673) (1.442, 7.86) (1.4413, 7.8563) knots -1 -1 -1 -1 -1 -1 -0.98571429 -0.97142857 -0.95714286 -0.94285714 -0.92857143 -0.91428571 -0.9 -0.88571429 -0.87142857 -0.85714286 -0.84285714 -0.82857143 -0.81428571 -0.8 -0.78571429 -0.77142857 -0.75714286 -0.74285714 -0.72857143 -0.71428571 -0.7 -0.68571429 -0.67142857 -0.65714286 -0.64285714 -0.62857143 -0.61428571 -0.6 -0.58571429 -0.57142857 -0.55714286 -0.54285714 -0.52857143 -0.51428571 -0.5 -0.48571429 -0.47142857 -0.45714286 -0.44285714 -0.42857143 -0.41428571 -0.4 -0.38571429 -0.37142857 -0.35714286 -0.34285714 -0.32857143 -0.31428571 -0.3 -0.28571429 -0.27142857 -0.25714286 -0.24285714 -0.22857143 -0.21428571 -0.2 -0.18571429 -0.17142857 -0.15714286 -0.14285714 -0.12857143 -0.11428571 -0.1 -0.08571429 -0.07142857 -0.05714286 -0.04285714 -0.02857143 -0.01428571 0 0 0 0 0 0
  arc A23 (0.9958, 7.5337) -> (1.4413, 7.8563) centre (1.0482, 7.9303) ccw
  arc A24 (0.9958, 7.5337) -> (0.988, 7.5348) centre (0, 0) ccw
  arc A25 (0.6411, 7.9617) -> (0.988, 7.5348) centre (1.04, 7.9314) ccw
  spline S12 degree 5 poles (0.6411, 7.9617) (0.6414, 7.9654) (0.6419, 7.9728) (0.6424, 7.9839) (0.6424, 7.9987) (0.6418, 8.0173) (0.6406, 8.0359) (0.6391, 8.0545) (0.6375, 8.0731) (0.6357, 8.0917) (0.6338, 8.1103) (0.6317, 8.129) (0.6294, 8.1476) (0.6268, 8.1663) (0.6239, 8.185) (0.6208, 8.2036) (0.6175, 8.2223) (0.6141, 8.241) (0.6105, 8.2597) (0.6068, 8.2783) (0.6029, 8.297) (0.5988, 8.3157) (0.5946, 8.3344) (0.5902, 8.3531) (0.5857, 8.3718) (0.581, 8.3904) (0.5761, 8.4091) (0.5711, 8.4278) (0.566, 8.4465) (0.5608, 8.4652) (0.5554, 8.4838) (0.5499, 8.5025) (0.5442, 8.5211) (0.5384, 8.5398) (0.5325, 8.5584) (0.5265, 8.5771) (0.5203, 8.5958) (0.514, 8.6145) (0.5076, 8.6331) (0.5011, 8.6517) (0.4944, 8.6703) (0.4876, 8.6888) (0.4807, 8.7073) (0.4737, 8.7258) (0.4666, 8.7445) (0.4593, 8.7632) (0.452, 8.782) (0.4445, 8.8008) (0.4369, 8.8194) (0.4292, 8.8377) (0.4214, 8.8558) (0.4136, 8.8737) (0.4056, 8.8918) (0.3974, 8.9103) (0.3891, 8.9293) (0.3807, 8.949) (0.3722, 8.9689) (0.3636, 8.9882) (0.3549, 9.0065) (0.3463, 9.0233) (0.3376, 9.0386) (0.3288, 9.0533) (0.3198, 9.0691) (0.3107, 9.0877) (0.3011, 9.1113) (0.291, 9.1417) (0.2805, 9.1804) (0.2692, 9.2285) (0.2574, 9.2868) (0.2448, 9.3557) (0.2316, 9.4356) (0.2204, 9.5085) (0.2117, 9.5681) (0.2058, 9.6101) (0.2028, 9.6316) knots 0 0 0 0 0 0 0.01428571 0.02857143 0.04285714 0.05714286 0.07142857 0.08571429 0.1 0.11428571 0.12857143 0.14285714 0.15714286 0.17142857 0.18571429 0.2 0.21428571 0.22857143 0.24285714 0.25714286 0.27142857 0.28571429 0.3 0.31428571 0.32857143 0.34285714 0.35714286 0.37142857 0.38571429 0.4 0.41428571 0.42857143 0.44285714 0.45714286 0.47142857 0.48571429 0.5 0.51428571 0.52857143 0.54285714 0.55714286 0.57142857 0.58571429 0.6 0.61428571 0.62857143 0.64285714 0.65714286 0.67142857 0.68571429 0.7 0.71428571 0.72857143 0.74285714 0.75714286 0.77142857 0.78571429 0.8 0.81428571 0.82857143 0.84285714 0.85714286 0.87142857 0.88571429 0.9 0.91428571 0.92857143 0.94285714 0.95714286 0.97142857 0.98571429 1 1 1 1 1 1
  arc A26 (0.2028, 9.6316) -> (-0.2028, 9.6316) centre (0, 0) ccw
  spline S13 degree 5 poles (-0.2028, 9.6316) (-0.2058, 9.6101) (-0.2117, 9.5681) (-0.2204, 9.5085) (-0.2316, 9.4356) (-0.2448, 9.3557) (-0.2574, 9.2868) (-0.2692, 9.2285) (-0.2805, 9.1804) (-0.291, 9.1417) (-0.3011, 9.1113) (-0.3107, 9.0877) (-0.3198, 9.0691) (-0.3288, 9.0533) (-0.3376, 9.0386) (-0.3463, 9.0233) (-0.3549, 9.0065) (-0.3636, 8.9882) (-0.3722, 8.9689) (-0.3807, 8.949) (-0.3891, 8.9293) (-0.3974, 8.9103) (-0.4056, 8.8918) (-0.4136, 8.8737) (-0.4214, 8.8558) (-0.4292, 8.8377) (-0.4369, 8.8194) (-0.4445, 8.8008) (-0.452, 8.782) (-0.4593, 8.7632) (-0.4666, 8.7445) (-0.4737, 8.7258) (-0.4807, 8.7073) (-0.4876, 8.6888) (-0.4944, 8.6703) (-0.5011, 8.6517) (-0.5076, 8.6331) (-0.514, 8.6145) (-0.5203, 8.5958) (-0.5265, 8.5771) (-0.5325, 8.5584) (-0.5384, 8.5398) (-0.5442, 8.5211) (-0.5499, 8.5025) (-0.5554, 8.4838) (-0.5608, 8.4652) (-0.566, 8.4465) (-0.5711, 8.4278) (-0.5761, 8.4091) (-0.581, 8.3904) (-0.5857, 8.3718) (-0.5902, 8.3531) (-0.5946, 8.3344) (-0.5988, 8.3157) (-0.6029, 8.297) (-0.6068, 8.2783) (-0.6105, 8.2597) (-0.6141, 8.241) (-0.6175, 8.2223) (-0.6208, 8.2036) (-0.6239, 8.185) (-0.6268, 8.1663) (-0.6294, 8.1476) (-0.6317, 8.129) (-0.6338, 8.1103) (-0.6357, 8.0917) (-0.6375, 8.0731) (-0.6391, 8.0545) (-0.6406, 8.0359) (-0.6418, 8.0173) (-0.6424, 7.9987) (-0.6424, 7.9839) (-0.6419, 7.9728) (-0.6414, 7.9654) (-0.6411, 7.9617) knots -1 -1 -1 -1 -1 -1 -0.98571429 -0.97142857 -0.95714286 -0.94285714 -0.92857143 -0.91428571 -0.9 -0.88571429 -0.87142857 -0.85714286 -0.84285714 -0.82857143 -0.81428571 -0.8 -0.78571429 -0.77142857 -0.75714286 -0.74285714 -0.72857143 -0.71428571 -0.7 -0.68571429 -0.67142857 -0.65714286 -0.64285714 -0.62857143 -0.61428571 -0.6 -0.58571429 -0.57142857 -0.55714286 -0.54285714 -0.52857143 -0.51428571 -0.5 -0.48571429 -0.47142857 -0.45714286 -0.44285714 -0.42857143 -0.41428571 -0.4 -0.38571429 -0.37142857 -0.35714286 -0.34285714 -0.32857143 -0.31428571 -0.3 -0.28571429 -0.27142857 -0.25714286 -0.24285714 -0.22857143 -0.21428571 -0.2 -0.18571429 -0.17142857 -0.15714286 -0.14285714 -0.12857143 -0.11428571 -0.1 -0.08571429 -0.07142857 -0.05714286 -0.04285714 -0.02857143 -0.01428571 0 0 0 0 0 0
  arc A27 (-0.988, 7.5348) -> (-0.6411, 7.9617) centre (-1.04, 7.9314) ccw
  arc A28 (-0.988, 7.5348) -> (-0.9958, 7.5337) centre (0, 0) ccw
  arc A29 (-1.4413, 7.8563) -> (-0.9958, 7.5337) centre (-1.0482, 7.9303) ccw